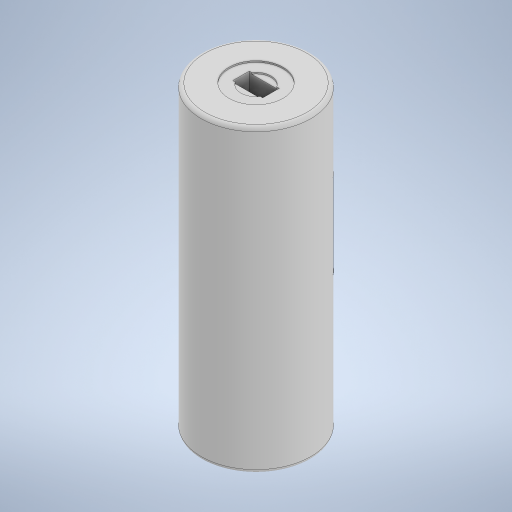
# Autodesk Inventor part: spinny
Saved by Autodesk Inventor 2024.2 (Build 282272000, 272)
## iProperties
Created: 2024-02-24
Part Number: spinny
Material: Generic
Document SubType Name: Modeling
Designer: Luke
Density: 1 g/cm^3
Appearance: Default
Author: Luke
Autodesk Inventor part; units mm, degrees
ref_plane "YZ Plane" through (0, 0, 0) normal (1, 0, 0) x (0, 1, 0)
ref_plane "XZ Plane" through (0, 0, 0) normal (0, 1, 0) x (-1, 0, 0)
ref_plane "XY Plane" through (0, 0, 0) normal (0, 0, 1) x (1, 0, 0)
sketch "Sketch1" plane through (0, 0, 0) normal (0, 1, 0) x (-1, 0, 0)
  circle A0 centre (0, 0) radius 9.271
  dimension "d0" = 18.542
  constraints: 1 centre point, 1 coincident
  measures "d0" diameter of A0
extrude "Extrusion1" add sketch "Sketch1" along normal blind 50.8
sketch "Sketch2" plane through (0, 50.8, 0) normal (0, 1, 0) x (1, 0, 0)
  line L0 (-2.54, 1.397) -> (2.54, 1.397)
  line L1 (2.54, 1.397) -> (2.54, -1.397)
  line L2 (2.54, -1.397) -> (-2.54, -1.397)
  line L3 (-2.54, -1.397) -> (-2.54, 1.397)
  line L4 (-2.54, 1.397) -> (2.54, -1.397) construction
  line L5 (2.54, 1.397) -> (-2.54, -1.397) construction
  point P0 (0, 0)
  point P1 (2.54, 0)
  point P2 (-2.54, 0)
  dimension "d3" = 2.794
  dimension "d4" = 5.08
  constraints: 12 end point, 4 midpoint, 2 parallel, 1 horizontal, 1 perpendicular
  measures "d3" distance between parallel lines of L0 L2
  measures "d4" distance of point (2.54, 0) point (-2.54, 0)
extrude "Extrusion2" cut sketch "Sketch2" against normal blind 12.7
fillet "Fillet2" radius 0.635 2 edges at (9.271, 50.8, 0) (9.271, 0, 0)
sketch "Sketch3" plane through (2.54, 38.1, 1.397) normal (0, 0, -1) x (-1, 0, 0)
  line L0 (9.652, -0.635) -> (-4.572, -0.635)
  line L1 (-4.572, -0.635) -> (-4.572, -14.859)
  line L2 (-4.572, -14.859) -> (9.652, -14.859)
  line L3 (9.652, -14.859) -> (9.652, -0.635)
  line L4 (9.652, -0.635) -> (-4.572, -14.859) construction
  line L5 (-4.572, -0.635) -> (9.652, -14.859) construction
  line L6 (11.811, 12.065) -> (-6.731, 12.065) projected
  point P0 (2.54, -38.1)
  point P1 (2.54, -7.747)
  dimension "d9" = 14.224
  dimension "d10" = 14.224
  dimension "d11" = 12.7
  constraints: 12 end point, 2 midpoint, 2 parallel, 1 horizontal, 1 perpendicular
  measures "d9" distance of L2.end L1.end
  measures "d10" distance of L1.end L0.end
  measures "d11" distance between parallel lines of L6 L0
extrude "Extrusion3" add sketch "Sketch3" along normal blind 127
sketch "Sketch4" plane through (2.54, 38.1, -125.603) normal (0, 0, -1) x (-1, 0, 0)
  line L0 (9.652, -0.635) -> (-4.572, -0.635) projected
  line L1 (-4.572, -14.859) -> (9.652, -14.859) projected
  line L2 (9.652, -0.635) -> (-4.572, -0.635)
  line L3 (-4.572, -0.635) -> (-4.572, -14.859)
  line L4 (-4.572, -14.859) -> (9.652, -14.859)
  line L5 (9.652, -14.859) -> (9.652, -0.635)
  point P0 (2.54, -38.1)
  point P1 (-4.572, -0.635)
  constraints: 8 end point, 2 parallel, 1 horizontal, 1 perpendicular
extrude "Extrusion4" cut sketch "Sketch4" against normal blind 127
sketch "Sketch5" plane through (0, 50.8, 0) normal (0, 1, 0) x (1, 0, 0)
  circle A0 centre (0, 0) radius 2.54
  dimension "d16" = 5.08
  constraints: 1 centre point, 1 coincident
  measures "d16" diameter of A0
extrude "Extrusion5" cut sketch "Sketch5" against normal blind 0.508
sketch "Sketch6" plane through (0, 50.8, 0) normal (0, 1, 0) x (1, 0, 0)
  arc A0 (-2.1213, -1.397) -> (2.1213, -1.397) centre (0, 0) ccw projected
  circle A1 centre (0, 0) radius 4.572
  dimension "d19" = 9.144
  constraints: 1 centre point, 1 coincident
  measures "d19" diameter of A1
extrude "Extrusion6" cut sketch "Sketch6" against normal blind 0.254
body "Solid1"
